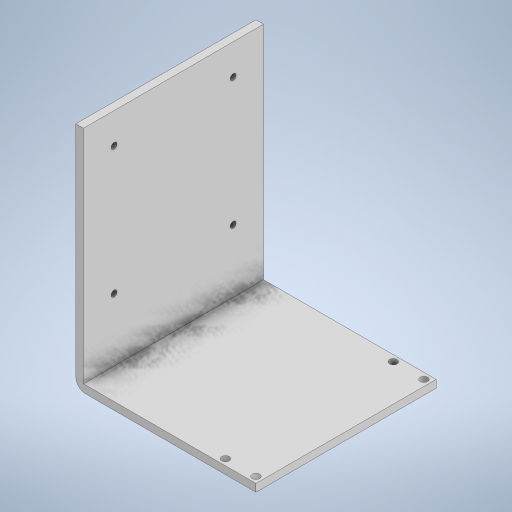
# Autodesk Inventor part: ConnectionBarcket(H)
Saved by Autodesk Inventor 2023 (Build 270158030, 158C)
## iProperties
Created: 2023-03-04
Part Number: ConnectionBarcket(H)
Material: Generic
Document SubType Name: Modeling
Designer: mpino
Density: 1 g/cm^3
Appearance: Default
Author: mpino
Autodesk Inventor part; units mm, degrees
ref_plane "YZ Plane" through (0, 0, 0) normal (1, 0, 0) x (0, 1, 0)
ref_plane "XZ Plane" through (0, 0, 0) normal (0, 1, 0) x (-1, 0, 0)
ref_plane "XY Plane" through (0, 0, 0) normal (0, 0, 1) x (1, 0, 0)
sketch "Sketch1" plane through (0, 0, 0) normal (0, 1, 0) x (-1, 0, 0)
  circle A0 centre (0, 0) radius 3.175
  line L0 (0, 0) -> (0, -139.7)
  circle A1 centre (0, -139.7) radius 3.175
  line L1 (0, 0) -> (-25.4, 0)
  circle A2 centre (-25.4, 0) radius 3.175
  line L2 (-25.4, 0) -> (-25.4, -139.7)
  circle A3 centre (-25.4, -139.7) radius 3.175
  line L3 (0, 0) -> (0, 5.08)
  line L4 (0, 5.08) -> (5.08, 5.08)
  line L5 (-25.4, -139.7) -> (-25.4, -144.78)
  line L6 (-25.4, -144.78) -> (-30.48, -144.78)
  line L7 (5.08, 5.08) -> (-30.48, 5.08)
  line L8 (-30.48, 5.08) -> (-30.48, -144.78)
  line L9 (-30.48, -144.78) -> (5.08, -144.78)
  line L10 (5.08, -144.78) -> (5.08, 5.08)
  dimension "d0" = 6.35
  dimension "d1" = 139.7
  dimension "d2" = 6.35
  dimension "d3" = 25.4
  dimension "d4" = 6.35
  dimension "d5" = 139.7
  dimension "d6" = 6.35
  dimension "d7" = 5.08
  dimension "d8" = 5.08
  dimension "d9" = 5.08
  dimension "d10" = 5.08
  constraints: 22 end point, 4 centre point, 4 coincident, 4 vertical, 3 horizontal, 2 parallel, 2 perpendicular
  measures "d0" diameter of A0
  measures "d1" distance of L0.start L0.end
  measures "d2" diameter of A1
  measures "d3" distance of L0.start L1.end
  measures "d4" diameter of A2
  measures "d5" distance of L2.start L2.end
  measures "d6" diameter of A3
  measures "d7" distance of L0.start L3.end
  measures "d8" distance of L3.end L4.end
  measures "d9" distance of L5.start L5.end
  measures "d10" distance of L5.end L6.end
extrude "Extrusion1" add sketch "Sketch1" along normal blind 6.35 contours A0 L3 L4 L10 L9 L5 A3 L2 A2 L1 | A0 L1 A2 L2 A3 L5 L6 L8 L7 L3
sketch "Sketch3" plane through (-5.08, 0, -144.78) normal (-1, 0, 0) x (0, 0, 1)
  line L0 (0, 6.35) -> (149.86, 6.35) projected
  line L1 (0, 0) -> (149.86, 0) projected
  line L2 (0, 6.35) -> (149.86, 6.35)
  line L3 (149.86, 6.35) -> (149.86, 0)
  line L4 (149.86, 0) -> (0, 0)
  line L5 (0, 0) -> (0, 6.35)
  point P0 (144.78, 0)
  constraints: 8 end point, 2 parallel, 1 horizontal, 1 perpendicular
extrude "Extrusion3" add sketch "Sketch3" along normal blind 114.3
sketch "Sketch4" plane through (0, 6.35, 0) normal (0, 1, 0) x (1, 0, 0)
  line L0 (30.48, 144.78) -> (-119.38, 144.78) projected
  line L1 (30.48, -5.08) -> (-119.38, -5.08) projected
  line L2 (-119.38, 144.78) -> (-113.03, 144.78)
  line L3 (-113.03, 144.78) -> (-113.03, -5.08)
  line L4 (-113.03, -5.08) -> (-119.38, -5.08)
  line L5 (-119.38, -5.08) -> (-119.38, 144.78)
  point P0 (0, 0)
  point P1 (-119.38, -5.08)
  dimension "d19" = 6.35
  constraints: 8 end point, 2 parallel, 1 horizontal, 1 perpendicular, 1 point on line
  measures "d19" distance of L3.end L4.end
extrude "Extrusion4" add sketch "Sketch4" along normal blind 184.15
fillet "Fillet1" radius 7.9375 1 edges at (-119.38, 0, -69.85)
sketch "Sketch5" plane through (-119.38, 0, -144.78) normal (-1, 0, 0) x (0, 0, 1)
  line L0 (149.86, 190.5) -> (0, 190.5) projected
  line L1 (0, 190.5) -> (25.4, 190.5)
  line L2 (25.4, 190.5) -> (25.4, 165.1)
  line L3 (149.86, 190.5) -> (124.46, 190.5)
  line L4 (124.46, 190.5) -> (124.46, 165.1)
  line L5 (0, 7.9375) -> (25.4, 7.9375)
  line L6 (149.86, 7.9375) -> (0, 7.9375) projected
  line L7 (25.4, 7.9375) -> (25.4, 58.7375)
  line L8 (149.86, 7.9375) -> (124.46, 7.9375)
  line L9 (124.46, 7.9375) -> (124.46, 58.7375)
  point P0 (144.78, 0)
  dimension "d23" = 25.4
  dimension "d24" = 25.4
  dimension "d25" = 25.4
  dimension "d26" = 25.4
  dimension "d27" = 25.4
  dimension "d29" = 50.8
  dimension "d30" = 25.4
  dimension "d31" = 50.8
  dimension "d32" = 90
  constraints: 16 end point, 3 point on line, 3 vertical, 1 perpendicular
  measures "d23" distance of L0.end L1.end
  measures "d24" distance of L1.end L2.end
  measures "d25" distance of L0.start L3.end
  measures "d26" distance of L3.end L4.end
  measures "d27" distance of L5.start L5.end
  measures "d29" distance of L5.end L7.end
  measures "d30" distance of L6.start L8.end
  measures "d31" distance of L8.end L9.end
  measures "d32" angle of L5 L4
hole "Hole1" at (-119.38, 165.1, -119.38) at (-119.38, 165.1, -20.32) at (-119.38, 58.7375, -119.38) at (-119.38, 58.7375, -20.32) direction (1, 0, 0) diameter 4.9784 depth 19.05 tip angle 118 thread size "1/4-20 UNC" class "2B" standard "ANSI Unified Screw Threads"
body "Solid1"
